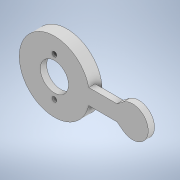
# Autodesk Inventor part: motor_holder_1
Saved by Autodesk Inventor 2020 (Build 240168000, 168)
## iProperties
Created: 2019-10-15
Part Number: motor_holder_1
Material: Generic
Document SubType Name: Modeling
Designer: psrob
Density: 1 g/cm^3
Appearance: Default
Author: psrob
Autodesk Inventor part; units mm, degrees
ref_plane "YZ Plane" through (0, 0, 0) normal (1, 0, 0) x (0, 1, 0)
ref_plane "XZ Plane" through (0, 0, 0) normal (0, 1, 0) x (-1, 0, 0)
ref_plane "XY Plane" through (0, 0, 0) normal (0, 0, 1) x (1, 0, 0)
sketch "Sketch1" plane through (0, 0, 0) normal (0, 0, 1) x (1, 0, 0)
  circle A0 centre (10.5, -10.5) radius 1 projected
  circle A1 centre (10.5, 10.5) radius 1 projected
  circle A2 centre (-10.5, -10.5) radius 1 projected
  circle A3 centre (-10.5, 10.5) radius 1 projected
  circle A4 centre (0, -12.5) radius 1.5 projected
  circle A5 centre (0, 12.5) radius 1.5 projected
  circle A6 centre (0, 0) radius 6.5 projected
  circle A7 centre (0, 0) radius 18 projected
  circle A8 centre (0, 0) radius 9
  circle A9 centre (0, 0) radius 18
  dimension "d0" = 18
  dimension "d1" = 36
  constraints: 2 centre point, 2 coincident
  measures "d0" diameter of A8
  measures "d1" diameter of A9
extrude "Extrusion1" add sketch "Sketch1" along normal blind 4 contours A0 | A1 | A2 | A3 | A7
sketch "Sketch2" plane through (0, 0, 4) normal (0, 0, 1) x (1, 0, 0)
  circle A0 centre (0, 0) radius 18 projected
  circle A1 centre (0, -12.5) radius 1.5 projected
  circle A2 centre (0, 12.5) radius 1.5 projected
  circle A3 centre (0, 0) radius 9 projected
  line L0 (0, 18) -> (40, 18)
  line L1 (40, 18) -> (40, -18)
  line L2 (40, -18) -> (0, -18)
  line L3 (0, -18) -> (0, 18)
  line L4 (0, 0) -> (0, 18)
  point P0 (0, -18)
  dimension "d4" = 40
  dimension "d5" = 36
  constraints: 10 end point, 2 parallel, 1 horizontal, 1 perpendicular, 1 vertical, 2 other
  measures "d4" distance of L1.end L2.end
  measures "d5" distance of L0.end L1.end
extrude "Extrusion2" add sketch "Sketch2" against normal blind 4 contours A0 L0 L1 L2
sketch "Sketch3" plane through (0, 0, 0) normal (0, 0, -1) x (-1, 0, 0)
  line L0 (0, 18) -> (-40, 18) projected
  line L1 (-40, 18) -> (-40, -18) projected
  line L2 (-40, -18) -> (0, -18) projected
  arc A0 (0, -18) -> (0, 18) centre (0, 0) ccw projected
  circle A1 centre (0, -12.5) radius 1.5 projected
  circle A2 centre (0, 12.5) radius 1.5 projected
  circle A3 centre (0, 0) radius 9 projected
  circle A4 centre (0, 0) radius 18
  circle A5 centre (0, 0) radius 20
  point P0 (-8.7178, 18)
  point P1 (-8.7178, -18)
  dimension "d8" = 36
  dimension "d9" = 40
  constraints: 2 centre point, 2 coincident
  measures "d8" diameter of A4
  measures "d9" diameter of A5
extrude "Extrusion3" add sketch "Sketch3" against normal blind 4 contours L0 A5 L2 A0
sketch "Sketch4" plane through (0, 0, 0) normal (0, 0, -1) x (-1, 0, 0)
  line L0 (-8.7178, 18) -> (-40, 18) projected
  line L1 (-40, 18) -> (-40, -18) projected
  line L2 (-40, -18) -> (-8.7178, -18) projected
  arc A0 (-8.7178, -18) -> (-8.7178, 18) centre (0, 0) ccw projected
  circle A1 centre (0, -12.5) radius 1.5 projected
  circle A2 centre (0, 12.5) radius 1.5 projected
  circle A3 centre (0, 0) radius 9 projected
  circle A4 centre (0, 0) radius 20
  circle A5 centre (0, 0) radius 22.5
  dimension "d12" = 40
  dimension "d13" = 45
  constraints: 2 centre point, 2 coincident
  measures "d12" diameter of A4
  measures "d13" diameter of A5
extrude "Extrusion4" add sketch "Sketch4" along normal mid plane 8 contours A4 L2 A5 L0 | L0 A5 L2 A0
sketch "Sketch5" plane through (0, 0, 0) normal (0, 0, -1) x (-1, 0, 0)
  arc A0 (-13.5, 18) -> (-13.5, -18) centre (0, 0) ccw projected
  line L0 (-13.5, 18) -> (-40, 18) projected
  line L1 (-40, 18) -> (-40, -18) projected
  line L2 (-40, -18) -> (-13.5, -18) projected
  line L3 (-40, 18) -> (-40, -18) projected
  line L4 (-40, 0) -> (-22.5, 0)
  line L5 (-58.0626, -5) -> (-58.0626, 5)
  line L6 (-58.0626, 5) -> (-21.9374, 5)
  line L7 (-21.9374, 5) -> (-21.9374, -5)
  line L8 (-21.9374, -5) -> (-58.0626, -5)
  line L9 (-58.0626, -5) -> (-21.9374, 5) construction
  line L10 (-58.0626, 5) -> (-21.9374, -5) construction
  circle A1 centre (0, 0) radius 22.5 projected
  point P0 (-40, 5)
  point P1 (-40, -5)
  dimension "d16" = 10
  constraints: 14 end point, 3 midpoint, 3 point on circle, 2 parallel, 1 perpendicular
  measures "d16" distance of L5.start L5.end
extrude "Extrusion5" cut sketch "Sketch5" against normal blind 8 contours A0 L6 L1 L0 | A0 L2 L1 L8
sketch "Sketch6" plane through (0, 0, 0) normal (0, 0, -1) x (-1, 0, 0)
  line L0 (-21.9374, 5) -> (-40, 5) projected
  line L1 (-40, 5) -> (-40, -5) projected
  line L2 (-40, -5) -> (-21.9374, -5) projected
  arc A0 (-21.9374, 5) -> (-21.9374, -5) centre (0, 0) ccw projected
  line L3 (0, 0) -> (-50, 0)
  circle A1 centre (-50, 0) radius 10
  line L4 (-40, 5) -> (-40, -5) projected
  line L5 (-40, 5) -> (-44, 8)
  line L6 (-40, -5) -> (-44, -8)
  line L7 (-50, 0) -> (-44, -8)
  line L8 (-50, 0) -> (-44, 8)
  dimension "d19" = 50
  dimension "d20" = 20
  constraints: 10 end point, 2 perpendicular, 2 point on circle, 1 centre point, 1 coincident, 1 horizontal
  measures "d19" distance of L3.start L3.end
  measures "d20" diameter of A1
extrude "Extrusion6" add sketch "Sketch6" against normal up to surface (4 mm away) contours L1 A1 L5 | A1 L7 L3 | L3 L8 A1 | L1 L6 A1 | L8 L7 A1
body "Solid1"
